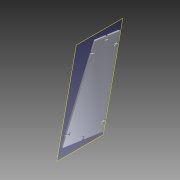
# Autodesk Inventor part: Panel_side
Saved by Autodesk Inventor 2013 (Build 170138000, 138)
## iProperties
Created: 2013-02-02
Part Number: Panel_side
Material: Aluminum 6061
Document SubType Name: Modeling
Designer: xylzlyx
Density: 1 g/cm^3
ScrewLen: 0.500 in
ScrewHoleD: 0.150 in
NutFlatsGap: 0.323 in
NutHeightGap: 0.119 in
SlotFilletRad: 0.020 in
ScrewHoleDist: 1.000 in
Author: xylzlyx
Autodesk Inventor part; units mm, degrees
ref_plane "YZ Plane" through (0, 0, 0) normal (1, 0, 0) x (0, 1, 0)
ref_plane "XZ Plane" through (0, 0, 0) normal (0, 1, 0) x (-1, 0, 0)
ref_plane "XY Plane" through (0, 0, 0) normal (0, 0, 1) x (1, 0, 0)
ref_plane "Work Plane1" through (-221.4413, -90.9255, -118.1004) normal (-0.9848078, 0.1736482, 0) x (-0.1736482, -0.9848078, 0)
sketch "Sketch1" plane through (-221.4413, -90.9255, -118.1004) normal (-0.9848078, 0.1736482, 0) x (-0.1736482, -0.9848078, 0)
  line L0 (0, 0) -> (-0.5513, 3.1268) construction
  line L1 (-0.5513, 3.1268) -> (245.7896, 46.5633) construction
  line L2 (245.7896, 46.5633) -> (246.341, 43.4366) construction
  line L3 (246.341, 43.4366) -> (0, 0) construction
  line L4 (254.4978, -57.6752) -> (251.371, -58.2265) construction
  line L5 (251.371, -58.2265) -> (233.8339, 41.2312) construction
  line L6 (233.8339, 41.2312) -> (236.9607, 41.7826) construction
  line L7 (236.9607, 41.7826) -> (254.4978, -57.6752) construction
  line L8 (12.5071, 2.2053) -> (23.1628, -58.2265) construction
  line L9 (23.1628, -58.2265) -> (20.0361, -58.7779) construction
  line L10 (20.0361, -58.7779) -> (9.3803, 1.654) construction
  line L11 (9.3803, 1.654) -> (12.5071, 2.2053) construction
  line L12 (264.2669, -61.4015) -> (10.2669, -61.4015) construction
  line L13 (10.2669, -61.4015) -> (10.2669, -58.2265) construction
  line L14 (10.2669, -58.2265) -> (264.2669, -58.2265) construction
  line L15 (264.2669, -58.2265) -> (264.2669, -61.4015) construction
  line L16 (233.8339, 41.2312) -> (251.371, -58.2265)
  line L17 (251.371, -58.2265) -> (23.1628, -58.2265)
  line L18 (23.1628, -58.2265) -> (12.5071, 2.2053)
  line L19 (12.5071, 2.2053) -> (233.8339, 41.2312)
  point P0 (-127.997, 118.1004)
  constraints: 40 end point, 4 collinear, 2 horizontal, 2 vertical, 28 other
extrude "SidePanel" add sketch "Sketch1" against normal blind 3.175
fillet "CornerFillet" radius 1 4 edges at (-263.5281, -338.7532, -176.327) (-260.4828, -321.4826, -76.8692) (-223.9001, -114.0121, -176.327) (-222.0498, -103.5182, -115.8951)
sketch "ScrewSketch" plane through (-221.4413, -90.9255, -118.1004) normal (-0.9848078, 0.1736482, 0) x (0, 0, 1)
  line L0 (-57.0529, -251.164) -> (40.2464, -234.0076) projected
  line L1 (41.0576, -232.8491) -> (2.379, -13.4919) projected
  line L2 (-61.4015, -11.2669) -> (-61.4015, -263.2669) projected
  line L3 (-58.2265, -250.1792) -> (-58.2265, -24.0019) projected
  line L4 (-61.4015, -226.6779) -> (-48.7015, -226.6779)
  line L5 (-61.4015, -222.8806) -> (-48.7015, -222.8806)
  line L6 (-61.4015, -222.8806) -> (-61.4015, -226.6779)
  line L7 (-48.7015, -226.6779) -> (-48.7015, -222.8806)
  line L8 (-61.4015, -47.5033) -> (-48.7015, -47.5033)
  line L9 (-48.7015, -47.5033) -> (-48.7015, -51.3006)
  line L10 (-48.7015, -51.3006) -> (-61.4015, -51.3006)
  line L11 (-61.4015, -51.3006) -> (-61.4015, -47.5033)
  line L12 (3.3004, -0.4335) -> (46.3897, -244.8048) projected
  line L13 (-2.9203, -38.2902) -> (9.5867, -36.0848)
  line L14 (-2.9203, -38.2902) -> (-2.261, -42.0298)
  line L15 (-2.261, -42.0298) -> (10.2461, -39.8245)
  line L16 (10.2461, -39.8245) -> (9.5867, -36.0848)
  line L17 (27.5963, -211.3588) -> (40.1034, -209.1535)
  line L18 (27.5963, -211.3588) -> (26.9369, -207.6192)
  line L19 (26.9369, -207.6192) -> (39.444, -205.4138)
  line L20 (39.444, -205.4138) -> (40.1034, -209.1535)
  line L21 (40.7978, -237.1343) -> (-56.6904, -254.3241) projected
  line L22 (0.6692, -9.5539) -> (-57.2417, -19.7652) projected
  line L23 (-48.7015, -228.875) -> (-48.7015, -220.6835)
  line L24 (-48.7015, -220.6835) -> (-51.7337, -220.6835)
  line L25 (-48.7015, -228.875) -> (-51.7337, -228.875)
  line L26 (-51.7337, -228.875) -> (-51.7337, -220.6835)
  line L27 (-48.7015, -45.3062) -> (-48.7015, -53.4977)
  line L28 (-48.7015, -53.4977) -> (-51.7337, -53.4977)
  line L29 (-51.7337, -53.4977) -> (-51.7337, -45.3062)
  line L30 (-51.7337, -45.3062) -> (-48.7015, -45.3062)
  line L31 (-1.8794, -44.1935) -> (-3.3019, -36.1265)
  line L32 (-1.8794, -44.1935) -> (1.1066, -43.667)
  line L33 (1.1066, -43.667) -> (-0.3158, -35.5999)
  line L34 (-0.3158, -35.5999) -> (-3.3019, -36.1265)
  line L35 (27.9778, -213.5225) -> (26.5554, -205.4555)
  line L36 (26.5554, -205.4555) -> (29.5415, -204.9289)
  line L37 (29.5415, -204.9289) -> (30.9639, -212.996)
  line L38 (30.9639, -212.996) -> (27.9778, -213.5225)
  line L39 (-6.0765, -245.3995) -> (-8.2819, -232.8925)
  line L40 (-12.0215, -233.5519) -> (-9.8161, -246.0589)
  line L41 (-8.2819, -232.8925) -> (-12.0215, -233.5519)
  line L42 (-6.0765, -245.3995) -> (-9.8161, -246.0589)
  line L43 (-14.1852, -233.9334) -> (-6.1181, -232.5109)
  line L44 (-13.6587, -236.9194) -> (-14.1852, -233.9334)
  line L45 (-13.6587, -236.9194) -> (-5.5916, -235.497)
  line L46 (-5.5916, -235.497) -> (-6.1181, -232.5109)
  line L47 (-26.4165, -14.3299) -> (-24.2111, -26.8369)
  line L48 (-24.2111, -26.8369) -> (-27.9507, -27.4963)
  line L49 (-27.9507, -27.4963) -> (-30.1561, -14.9893)
  line L50 (-30.1561, -14.9893) -> (-26.4165, -14.3299)
  line L51 (-30.1145, -27.8778) -> (-22.0474, -26.4554)
  line L52 (-22.0474, -26.4554) -> (-22.5739, -23.4694)
  line L53 (-22.5739, -23.4694) -> (-30.641, -24.8918)
  line L54 (-30.641, -24.8918) -> (-30.1145, -27.8778)
  line L55 (-61.4015, -224.7792) -> (-48.7015, -224.7792) construction
  line L56 (-61.4015, -49.4019) -> (-48.7015, -49.4019) construction
  line L57 (9.9164, -37.9547) -> (-2.5907, -40.16) construction
  line L58 (39.7737, -207.2836) -> (27.2666, -209.489) construction
  point P0 (-7.9463, -245.7292)
  point P1 (-10.1517, -233.2222)
  point P2 (-28.2863, -14.6596)
  point P3 (-26.0809, -27.1666)
  dimension "d7" = 12.7
  dimension "d8" = 3.7973
  dimension "d10" = 12.7
  dimension "d11" = 3.7973
  dimension "d14" = 12.7
  dimension "d17" = 3.7973
  dimension "d18" = 12.7
  dimension "d20" = 3.7973
  dimension "d21" = 8.1915
  dimension "d22" = 3.0321
  dimension "d23" = 8.1915
  dimension "d24" = 3.0321
  dimension "d25" = 8.1915
  dimension "d26" = 3.0321
  dimension "d27" = 8.1915
  dimension "d28" = 3.0321
  dimension "d29" = 12.7
  dimension "d30" = 3.7973
  dimension "d31" = 8.1915
  dimension "d32" = 3.0321
  dimension "d33" = 3.7973
  dimension "d34" = 12.7
  dimension "d35" = 8.1915
  dimension "d36" = 3.0321
  dimension "d40" = 25.4
  dimension "d41" = 25.4
  dimension "d42" = 25.4
  dimension "d43" = 25.4
  constraints: 104 end point, 39 parallel, 16 midpoint, 9 collinear, 6 perpendicular, 6 point on line
  measures "d7" distance of L4.start L4.end
  measures "d8" distance between parallel lines of L4 L5
  measures "d10" distance of L8.start L8.end
  measures "d11" distance of L10.end L8.start
  measures "d14" distance of L13.start L13.end
  measures "d17" distance between parallel lines of L13 L15
  measures "d18" distance of L17.start L17.end
  measures "d20" distance of L19.end L17.end
  measures "d21" distance of L23.start L23.end
  measures "d22" distance of L23.end L24.end
  measures "d23" distance of L27.start L27.end
  measures "d24" distance of L27.end L28.end
  measures "d25" distance of L31.start L31.end
  measures "d26" distance of L31.start L32.end
  measures "d27" distance of L35.start L35.end
  measures "d28" distance of L35.end L36.end
  measures "d29" distance of L39.start L39.end
  measures "d30" distance of L39.end L40.start
  measures "d31" distance of L43.start L43.end
  measures "d32" distance of L44.start L43.start
  measures "d33" distance of L49.end L47.start
  measures "d34" distance of L48.end L49.end
  measures "d35" distance of L51.start L51.end
  measures "d36" distance of L51.end L52.end
  measures "d40" vertical distance of L55.start L3.start
  measures "d41" vertical distance of L3.end L56.start
  measures "d42" distance from line of L1.end L57
  measures "d43" distance from line of L1.start L58
extrude "ScrewSlots" cut sketch "ScrewSketch" against normal blind 25.4 contours L40 L45 L39 L0 | L0 L39 L21 L40 | L45 L44 L43 L40 | L40 L41 L39 L45 | L39 L43 L46 L45 | L17 L37 L19 L1 | L1 L19 L12 L17 | L37 L38 L35 L17 | L17 L18 L19 L37 | L15 L33 L13 L1 | L1 L13 L12 L15 | L19 L35 L36 L37 | L33 L32 L31 L15 | L15 L14 L13 L33 | L13 L31 L34 L33 | L8 L3 L10 L2 | L8 L29 L10 L3 | L5 L3 L4 L2 | L29 L30 L27 L8 | L8 L9 L10 L29 | L5 L26 L4 L3 | L10 L27 L28 L29 | L26 L24 L23 L5 | L5 L7 L4 L26 | L4 L23 L25 L26 | L47 L53 L49 L22 | L53 L52 L51 L47 | L47 L48 L49 L53 | L49 L51 L54 L53
fillet "SlotFillets" radius 0.5 48 edges at (-261.9482, -329.7932, -124.7283) (-260.8378, -323.4961, -125.8558) (-262.0627, -330.4426, -128.4679) (-260.9523, -324.1455, -129.5954) (-261.0186, -324.5212, -131.7591) (-260.5001, -321.5805, -132.2856) (-260.2531, -320.1797, -124.2186) (-260.7716, -323.1204, -123.6921) (-256.4886, -298.8304, -87.5181) (-256.8643, -300.9612, -87.1365) (-256.9558, -301.4797, -90.1226) (-255.5549, -293.5352, -91.545) (-255.4635, -293.0167, -88.559) (-255.8392, -295.1476, -88.1775) (-256.2928, -297.72, -81.1238) (-255.6434, -294.0372, -81.7832) (-259.6217, -316.599, -166.802) (-259.6217, -316.599, -169.8341) (-259.2402, -314.4353, -169.8341) (-259.2402, -314.4353, -176.327) (-258.5808, -310.6957, -176.327) (-258.5808, -310.6957, -169.8341) (-258.1992, -308.5319, -169.8341) (-258.1992, -308.5319, -166.802) (-229.1677, -143.8861, -166.802) (-229.1677, -143.8861, -169.8341) (-228.7862, -141.7223, -169.8341) (-228.7862, -141.7223, -176.327) (-228.1268, -137.9827, -176.327) (-228.1268, -137.9827, -169.8341) (-227.7453, -135.819, -169.8341) (-227.7453, -135.819, -166.802) (-224.7189, -118.6554, -148.2149) (-224.4719, -117.2546, -140.1479) (-223.9534, -114.3139, -140.6744) (-224.0196, -114.6897, -142.8381) (-224.1341, -115.339, -146.5777) (-224.2004, -115.7148, -148.7414) (-223.0238, -109.0419, -147.7052) (-222.9093, -108.3926, -143.9656) (-226.1513, -126.7787, -121.4023) (-227.4607, -134.2047, -116.9938) (-227.5521, -134.7232, -119.9799) (-226.0598, -126.2602, -118.4163) (-226.2398, -127.2807, -111.6405) (-226.8891, -130.9635, -110.9811) (-226.4356, -128.3911, -118.0347) (-227.0849, -132.0739, -117.3753)
equation "\"d7\" = ScrewLen"
equation "\"d8\" = ScrewHoleD"
equation "\"d10\" = ScrewLen"
equation "\"d11\" = ScrewHoleD"
equation "\"d14\" = ScrewLen"
equation "\"d17\" = ScrewHoleD"
equation "\"d18\" = ScrewLen"
equation "\"d20\" = ScrewHoleD"
equation "\"d21\" = NutFlatsGap"
equation "\"d22\" = NutHeightGap"
equation "\"d23\" = NutFlatsGap"
equation "\"d24\" = NutHeightGap"
equation "\"d25\" = NutFlatsGap"
equation "\"d26\" = NutHeightGap"
equation "\"d27\" = NutFlatsGap"
equation "\"d28\" = NutHeightGap"
equation "\"d29\" = ScrewLen"
equation "\"d30\" = ScrewHoleD"
equation "\"d31\" = NutFlatsGap"
equation "\"d32\" = NutHeightGap"
equation "\"d33\" = ScrewHoleD"
equation "\"d34\" = ScrewLen"
equation "\"d35\" = NutFlatsGap"
equation "\"d36\" = NutHeightGap"
equation "\"ScrewLen\" = 12.7"
equation "\"ScrewHoleD\" = 3.7973"
equation "\"NutFlatsGap\" = 8.1915"
equation "\"NutHeightGap\" = 3.03212"
equation "\"SlotFilletRad\" = 0.5"
equation "\"ScrewHoleDist\" = 25.4"
body "Solid1"
